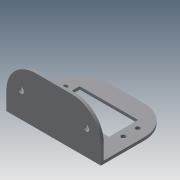
# Autodesk Inventor part: drzak_servo
Saved by Autodesk Inventor 2013 (Build 170138000, 138)
## iProperties
Created: 2013-05-13
Part Number: drzak_servo
Material: Generic
Document SubType Name: Modeling
Designer: idle-rug
Density: 1 g/cm^3
Author: idle-rug
Autodesk Inventor part; units mm, degrees
ref_plane "YZ Plane" through (0, 0, 0) normal (1, 0, 0) x (0, 1, 0)
ref_plane "XZ Plane" through (0, 0, 0) normal (0, 1, 0) x (-1, 0, 0)
ref_plane "XY Plane" through (0, 0, 0) normal (0, 0, 1) x (1, 0, 0)
sketch "Sketch1" plane through (0, 0, 0) normal (0, 1, 0) x (-1, 0, 0)
  line L0 (-32.5, -25) -> (32.5, -25)
  line L1 (32.5, -25) -> (32.5, 25)
  line L2 (32.5, 25) -> (-32.5, 25)
  line L3 (-32.5, 25) -> (-32.5, -25)
  line L4 (-32.5, -25) -> (32.5, 25) construction
  line L5 (32.5, -25) -> (-32.5, 25) construction
  point P0 (0, 0)
  dimension "d0" = 65
  dimension "d1" = 50
  constraints: 12 end point, 2 midpoint, 2 parallel, 1 horizontal, 1 perpendicular
  measures "d0" distance of L2.end L1.end
  measures "d1" distance of L1.end L0.end
extrude "Extrusion1" add sketch "Sketch1" along normal blind 2
sketch "Sketch2" plane through (0, 2, 0) normal (0, 1, 0) x (1, 0, 0)
  line L0 (32.5, -25) -> (32.5, 25) projected
  line L1 (-32.5, 25) -> (32.5, 25)
  line L2 (32.5, 25) -> (32.5, 23)
  line L3 (32.5, 23) -> (-32.5, 23)
  line L4 (-32.5, 23) -> (-32.5, 25)
  point P0 (0, 0)
  dimension "d4" = 2
  constraints: 8 end point, 2 parallel, 1 horizontal, 1 perpendicular, 1 point on line
  measures "d4" distance of L1.end L2.end
extrude "Extrusion2" add sketch "Sketch2" along normal blind 48
sketch "Sketch3" plane through (32.5, 0, -25) normal (0, 0, -1) x (-1, 0, 0)
  line L0 (0, 0) -> (0, 50) projected
  line L1 (32.5, 0) -> (32.5, 28)
  line L2 (52.6, 38) -> (12.4, 38)
  line L3 (12.4, 38) -> (12.4, 18)
  line L4 (12.4, 18) -> (52.6, 18)
  line L5 (52.6, 18) -> (52.6, 38)
  line L6 (52.6, 38) -> (12.4, 18) construction
  line L7 (12.4, 38) -> (52.6, 18) construction
  circle A0 centre (7.65, 32.95) radius 1.5
  circle A1 centre (7.65, 23.05) radius 1.5
  circle A2 centre (57.35, 32.95) radius 1.5
  circle A3 centre (57.35, 23.05) radius 1.5
  dimension "d10" = 28
  dimension "d11" = 40.2
  dimension "d12" = 20
  dimension "d15" = 3
  dimension "d16" = 3
  dimension "d18" = 3
  dimension "d20" = 3
  constraints: 14 end point, 4 centre point, 3 parallel, 2 midpoint, 1 horizontal, 1 perpendicular
  measures "d10" distance of L1.start L1.end
  measures "d11" distance of L4.end L3.end
  measures "d12" distance of L3.end L2.end
  measures "d15" diameter of A0
  measures "d16" diameter of A1
  measures "d18" diameter of A2
  measures "d20" diameter of A3
extrude "Extrusion3" cut sketch "Sketch3" against normal blind 2
sketch "Sketch4" plane through (-32.5, 0, 25) normal (0, 0, 1) x (1, 0, 0)
  line L0 (0, 0) -> (65, 0) projected
  line L1 (65, 0) -> (65, 2) projected
  line L2 (0, 2) -> (65, 2) projected
  line L3 (0, 0) -> (0, 2) projected
  point P0 (32.5, 0)
extrude "Extrusion4" cut sketch "Sketch4" against normal blind 17.4
fillet "Fillet1" radius 20 2 edges at (32.5, 50, -24) (-32.5, 50, -24)
fillet "Fillet2" radius 20 2 edges at (32.5, 1, 7.6) (-32.5, 1, 7.6)
sketch "Sketch5" plane through (0, 2, 0) normal (0, 1, 0) x (1, 0, 0)
  circle A0 centre (-22.5, 7.7) radius 2
  circle A1 centre (22.5, 7.7) radius 2
  point P0 (32.5, 23)
  point P1 (0, 0)
  dimension "d29" = 4
  dimension "d32" = 4
  constraints: 2 centre point
  measures "d29" diameter of A0
  measures "d32" diameter of A1
extrude "Extrusion5" cut sketch "Sketch5" against normal blind 2
body "Solid1"
